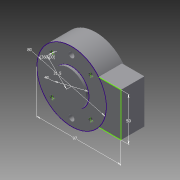
# Autodesk Inventor part: CFS080CA501U
Saved by Autodesk Inventor 2013 (Build 170138000, 138)
## iProperties
Created: 2013-01-30
Part Number: CFS080CA501U
Material: Generic
Document SubType Name: Modeling
Designer: Mahisorn
Density: 1 g/cm^3
Author: Mahisorn
Autodesk Inventor part; units mm, degrees
ref_plane "YZ Plane" through (0, 0, 0) normal (1, 0, 0) x (0, 1, 0)
ref_plane "XZ Plane" through (0, 0, 0) normal (0, 1, 0) x (-1, 0, 0)
ref_plane "XY Plane" through (0, 0, 0) normal (0, 0, 1) x (1, 0, 0)
sketch "Sketch1" plane through (0, 0, 0) normal (0, 1, 0) x (-1, 0, 0)
  circle A0 centre (0, 0) radius 40
  circle A1 centre (0, 0) radius 20
  line L0 (-57, 25) -> (-31.225, 25)
  line L1 (-31.225, -25) -> (-57, -25)
  line L2 (-57, -25) -> (-57, 25)
  point P0 (22.2739, 22.2739)
  point P1 (-22.2739, 22.2739)
  point P2 (-22.2739, -22.2739)
  point P3 (22.2739, -22.2739)
  dimension "d0" = 80
  dimension "d2" = 40
  dimension "d5" = 97
  dimension "d6" = 50
  dimension "d7" = 31.5
  dimension "d10" = 360
  constraints: 6 end point, 5 coincident, 2 centre point, 2 point on circle, 1 horizontal, 1 parallel, 7 other
  measures "d0" diameter of A0
  measures "d2" diameter of A1
  measures "d6" distance between parallel lines of L1 L0
  measures "d7" distance of point (22.274, 22.274) point (0, 0)
extrude "Extrusion1" add sketch "Sketch1" along normal blind 28 contours A0
extrude "Extrusion2" add sketch "Sketch1" along normal blind 28 contours A1
extrude "Extrusion3" add sketch "Sketch1" against normal blind 3 contours A1
extrude "Extrusion4" add sketch "Sketch1" along normal blind 27 contours A0 L1 L2 L0
hole "Hole1" at (-22.2739, 0, 22.2739) at (22.2739, 0, 22.2739) at (22.2739, 0, -22.2739) at (-22.2739, 0, -22.2739) direction (0, 1, 0) diameter 5.459 end through all thread size "M6x0.5" class "6H" standard "ANSI Metric M Profile"
sketch "Sketch2" plane through (0, 28, 0) normal (0, 1, 0) x (1, 0, 0)
  circle A0 centre (0, 0) radius 40 projected
  point P0 (0, 31.5)
  point P1 (0, -31.5)
  dimension "d27" = 31.5
  dimension "d30" = 360
  constraints: 3 other
  measures "d27" distance of A0.centre point (0, 31.5)
hole "Hole2" at (0, 28, 31.5) at (0, 28, -31.5) direction (0, -1, 0) diameter 6.6 end through all clearance for "Hex Head Bolt" size "M6" standard "Ansi Metric M Profile"
body "Solid1"
